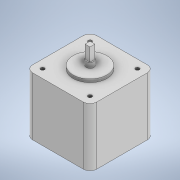
# Autodesk Inventor part: stepper
Saved by Autodesk Inventor 2020 (Build 240168000, 168)
## iProperties
Created: 2020-02-03
Part Number: stepper
Material: Generic
Document SubType Name: Modeling
Designer: Felix
Density: 1 g/cm^3
Appearance: Default
Author: Felix
Autodesk Inventor part; units mm, degrees
ref_plane "YZ Plane" through (0, 0, 0) normal (1, 0, 0) x (0, 1, 0)
ref_plane "XZ Plane" through (0, 0, 0) normal (0, 1, 0) x (-1, 0, 0)
ref_plane "XY Plane" through (0, 0, 0) normal (0, 0, 1) x (1, 0, 0)
sketch "Sketch1" plane through (0, 0, 0) normal (0, 1, 0) x (-1, 0, 0)
  line L0 (-16.5, -21) -> (16.5, -21)
  line L1 (21, -16.5) -> (21, 16.5)
  line L2 (16.5, 21) -> (-16.5, 21)
  line L3 (-21, 16.5) -> (-21, -16.5)
  line L4 (-21, -21) -> (21, 21) construction
  line L5 (21, -21) -> (-21, 21) construction
  arc A0 (21, 16.5) -> (16.5, 21) centre (16.5, 16.5) ccw
  arc A1 (-16.5, 21) -> (-21, 16.5) centre (-16.5, 16.5) ccw
  arc A2 (-21, -16.5) -> (-16.5, -21) centre (-16.5, -16.5) ccw
  arc A3 (16.5, -21) -> (21, -16.5) centre (16.5, -16.5) ccw
  point P0 (0, 0)
  dimension "d0" = 42
  dimension "d1" = 42
  dimension "d2" = 4.5
  constraints: 12 end point, 8 point on circle, 8 point on line, 8 tangent, 4 centre point, 3 equal radius, 2 midpoint, 2 parallel, 1 horizontal, 1 perpendicular
  measures "d0" distance of L5.end L4.end
  measures "d1" distance of L4.end L5.start
  measures "d2" radius of A0
extrude "Extrusion1" add sketch "Sketch1" along normal blind 38
sketch "Sketch2" plane through (0, 38, 0) normal (0, 1, 0) x (1, 0, 0)
  circle A0 centre (0, 0) radius 11
  dimension "d5" = 22
  constraints: 1 centre point, 1 coincident
  measures "d5" diameter of A0
extrude "Extrusion2" add sketch "Sketch2" along normal blind 2
sketch "Sketch3" plane through (0, 38, 0) normal (0, 1, 0) x (1, 0, 0)
  line L0 (-15.5, -15.5) -> (15.5, -15.5) construction
  line L1 (15.5, -15.5) -> (15.5, 15.5) construction
  line L2 (15.5, 15.5) -> (-15.5, 15.5) construction
  line L3 (-15.5, 15.5) -> (-15.5, -15.5) construction
  line L4 (-15.5, -15.5) -> (15.5, 15.5) construction
  line L5 (15.5, -15.5) -> (-15.5, 15.5) construction
  point P0 (0, 0)
  dimension "d8" = 31
  dimension "d9" = 31
  constraints: 12 end point, 4 coincident, 2 midpoint, 2 parallel, 1 horizontal, 1 perpendicular
  measures "d8" distance of L2.end L1.end
  measures "d9" distance of L1.end L0.end
hole "Hole1" at (-15.5, 38, 15.5) at (-15.5, 38, -15.5) at (15.5, 38, -15.5) at (15.5, 38, 15.5) direction (0, -1, 0) diameter 2.459 depth 6 thread size "M3x0.5" class "6H" standard "ISO Metric profile"
sketch "Sketch4" plane through (0, 40, 0) normal (0, 1, 0) x (1, 0, 0)
  circle A0 centre (0, 0) radius 2.5
  dimension "d17" = 5
  constraints: 1 centre point, 1 coincident
  measures "d17" diameter of A0
extrude "Extrusion3" add sketch "Sketch4" along normal blind 3.4
sketch "Sketch5" plane through (0, 43.4, 0) normal (0, 1, 0) x (1, 0, 0)
  line L0 (1.6, -1.6) -> (-1.6, -1.6)
  line L1 (-1.6, -1.6) -> (-1.6, 1.6)
  line L2 (-1.6, 1.6) -> (1.6, 1.6)
  line L3 (1.6, 1.6) -> (1.6, -1.6)
  circle A0 centre (0, 0) radius 2.5 construction
  line L4 (1.6, -1.6) -> (-1.6, 1.6) construction
  line L5 (-1.6, -1.6) -> (1.6, 1.6) construction
  circle A1 centre (0, 0) radius 2.5 construction
  circle A2 centre (0, 0) radius 11 projected
  dimension "d20" = 3.2
  dimension "d21" = 3.2
  constraints: 12 end point, 2 midpoint, 2 parallel, 1 horizontal, 1 perpendicular
  measures "d20" distance of L1.end L2.end
  measures "d21" distance of L0.end L1.end
extrude "Extrusion4" add sketch "Sketch5" along normal blind 8.6 contours L0 L1 L2 L3
body "Solid1"
